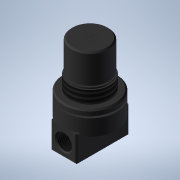
# Autodesk Inventor part: AP100-02_BODY
Saved by Autodesk Inventor 2021 (Build 250183000, 183)
## iProperties
Created: 2026-06-25
Part Number: AP100-02_BODY
Material: Generic
Catalog Web Link: www.3dfindit.com
Description: AP100 BODY-Pressure Control Valve
Vendor: SMC
Document SubType Name: Modeling
Designer: psAdmin
Manufacturer: SMC
Mass: 54.57 g
Surface Area: 113.774 cm^2
Volume: 54.57 cm^3
Density: 1 g/cm^3
Appearance: PSOLRGB-176-176-176
Category: PARTsolutions
Company: SMC
Title: AP100-02_BODY
Author: Cadenas PARTsolutions
Comments: Pressure Control Valve
PSOL_IDENT_0: {$CADENAS_DATA/23d-libs/smc_jp/air_line_equipment/pressure_control_equipment/pressure_control_valve/
PSOL_IDENT_1: parts/ap100_body.prj},187 {VTYP=3D},{NB=AP100-02_BODY},{LINA=AP100-02_BODY},{NN=AP100 BODY},{DATE=25
PSOL_IDENT_2: .06.2026 06:59:34},{GEOMDATE=28.10.2020 06:44:50},{VERSION=},{LINEID=10},{WBVAR=THREAD2,ACCESSORY},{
PSOL_IDENT_3: WBNUMERIC=}  {NB=AP100-02_BODY},{LINA=AP100-02_BODY},{KT=DUMMY},{THREAD2=02},{ACCESSORY=},{ORDER=AP1
PSOL_IDENT_4: 00-02},{RA=13.157},{RD=11.6}
NB: AP100-02_BODY
NN: AP100 BODY
NT: Pressure Control Valve
NBSYN: $ORDER._BODY
LINA: AP100-02_BODY
CATALOG: SMC (JP
THREAD2: (02) 1/4
ACCESSORY: (-) None
SUPPLIER: SMC
ARTICLENO: AP100-02_BODY
BOMINFO: AP100-02_BODY
CREATOR: CADENAS GmbH
Autodesk Inventor part; units mm, degrees
sketch "Sketch_1" plane through (0, 0, 0) normal (0, 0, 1) x (1, 0, 0)
  line L0 (-10, 10) -> (-10, -9)
  line L1 (-10, -9) -> (-9, -10)
  line L2 (-9, -10) -> (9, -10)
  line L3 (9, -10) -> (10, -9)
  line L4 (10, -9) -> (10, 10)
  line L5 (10, 10) -> (-10, 10)
  constraints: 12 end point
extrude "Extrusion1" add sketch "Sketch_1" along normal mid plane 40
sketch "Sketch_2" plane through (0, 0, 0) normal (0, 1, 0) x (-1, 0, 0)
  line L0 (15, 25) -> (-15, 25)
  line L1 (-15, 25) -> (-15, -25)
  line L2 (-15, -25) -> (15, -25)
  line L3 (15, -25) -> (15, 25)
  line L4 (10, -19) -> (10, 19)
  line L5 (10, 19) -> (9, 20)
  line L6 (9, 20) -> (-9, 20)
  line L7 (-9, 20) -> (-10, 19)
  line L8 (-10, 19) -> (-10, -19)
  line L9 (-10, -19) -> (-9, -20)
  line L10 (-9, -20) -> (9, -20)
  line L11 (9, -20) -> (10, -19)
  constraints: 24 end point
extrude "Extrusion2" cut sketch "Sketch_2" along normal mid plane 40
sketch "Sketch_3" plane through (0, 0, 0) normal (1, 0, 0) x (0, 1, 0)
  line L0 (15, 25) -> (-15, 25)
  line L1 (-15, 25) -> (-15, -25)
  line L2 (-15, -25) -> (15, -25)
  line L3 (15, -25) -> (15, -20)
  line L4 (15, -20) -> (-9, -20)
  line L5 (-9, -20) -> (-10, -19)
  line L6 (-10, -19) -> (-10, 19)
  line L7 (-10, 19) -> (-9, 20)
  line L8 (-9, 20) -> (15, 20)
  line L9 (15, 20) -> (15, 25)
  constraints: 20 end point
extrude "Extrusion3" cut sketch "Sketch_3" along normal mid plane 20
sketch "Sketch_4" plane through (0, 0, 0) normal (0, 0, 1) x (1, 0, 0)
  line L0 (0, 59) -> (0, 8)
  line L1 (0, 8) -> (-20, 8)
  line L2 (-20, 8) -> (-20, 20)
  line L3 (-20, 20) -> (-18, 20)
  line L4 (-18, 20) -> (-18, 21.5)
  line L5 (-18, 21.5) -> (-20, 21.5)
  line L6 (-20, 21.5) -> (-20, 24.5)
  line L7 (-20, 24.5) -> (-19, 25.5)
  line L8 (-19, 25.5) -> (-15, 25.5)
  line L9 (-15, 25.5) -> (-15, 35)
  line L10 (-15, 35) -> (-14, 35)
  line L11 (-14, 35) -> (-14, 36)
  line L12 (-14, 36) -> (-12, 36)
  line L13 (-12, 36) -> (-12, 37.09)
  line L14 (-12, 37.09) -> (-14, 37.09)
  line L15 (-14, 37.09) -> (-14, 58)
  line L16 (-14, 58) -> (-13, 59)
  line L17 (-13, 59) -> (0, 59)
  line L18 (0, 59) -> (0, 8)
  constraints: 38 end point
revolve "Revolution1" add sketch "Sketch_4" angle 360 about axis through (0, 59, 0) along (0, 1, 0)
thread "Thread1" size "M30x3.5" class "6g" standard "ISO Metric profile" full length
sketch "Sketch_5" plane through (0, 0, 0) normal (1, 0, 0) x (0, 1, 0)
  line L0 (0, 20) -> (0, 5.0961)
  line L1 (0, 5.0961) -> (-5.7225, 8.4)
  line L2 (-5.7225, 8.4) -> (-5.7225, 19.144)
  line L3 (-5.7225, 19.144) -> (-6.5785, 20)
  line L4 (-6.5785, 20) -> (0, 20)
  line L5 (0, 20) -> (0, 5.0961)
  constraints: 12 end point
revolve "Revolution2" cut sketch "Sketch_5" angle 360 about axis through (0, 0, 20) along (0, 0, 1)
thread "Thread2" size "G13.157x1.337" designation "G 1/4" standard "ISO Pipe Threads" full length
sketch "Sketch_6" plane through (0, 0, 0) normal (1, 0, 0) x (0, 1, 0)
  line L0 (0, -5.0961) -> (0, -20)
  line L1 (0, -20) -> (-6.5785, -20)
  line L2 (-6.5785, -20) -> (-5.7225, -19.144)
  line L3 (-5.7225, -19.144) -> (-5.7225, -8.4)
  line L4 (-5.7225, -8.4) -> (0, -5.0961)
  line L5 (0, -5.0961) -> (0, -20)
  constraints: 12 end point
revolve "Revolution3" cut sketch "Sketch_6" angle 360 about axis through (0, 0, -5.0961) along (0, 0, 1)
thread "Thread3" size "G13.157x1.337" designation "G 1/4" standard "ISO Pipe Threads" full length
sketch "Sketch_10" plane through (0, 59, 0) normal (0, 1, 0) x (1, 0, 0)
  line L0 (-3, -0.5) -> (-1, -0.5)
  arc A0 (-0.5, -1) -> (-1, -0.5) centre (-1, -1) ccw
  line L1 (-0.5, -1) -> (-0.5, -3)
  line L2 (-0.5, -3) -> (0.5, -3)
  line L3 (0.5, -3) -> (0.5, -1)
  arc A1 (1, -0.5) -> (0.5, -1) centre (1, -1) ccw
  line L4 (1, -0.5) -> (3, -0.5)
  line L5 (3, -0.5) -> (3, 0.5)
  line L6 (3, 0.5) -> (1, 0.5)
  arc A2 (0.5, 1) -> (1, 0.5) centre (1, 1) ccw
  line L7 (0.5, 1) -> (0.5, 3)
  line L8 (0.5, 3) -> (-0.5, 3)
  line L9 (-0.5, 3) -> (-0.5, 1)
  arc A3 (-1, 0.5) -> (-0.5, 1) centre (-1, 1) ccw
  line L10 (-1, 0.5) -> (-3, 0.5)
  line L11 (-3, 0.5) -> (-3, -0.5)
  constraints: 24 end point, 8 point on circle, 4 centre point
extrude "Extrusion4" cut sketch "Sketch_10" against normal blind 0.2
sketch "Sketch_11" plane through (0, 59, 0) normal (0, 1, 0) x (1, 0, 0)
  circle A0 centre (0, 0) radius 4.1
  circle A1 centre (0, 0) radius 4
  constraints: 2 centre point
extrude "Extrusion5" cut sketch "Sketch_11" against normal blind 1
ref_plane "body_dummy_XY" through (0, 0, 0) normal (0, 0, -1) x (1, 0, 0)
ref_plane "body_dummy_YZ" through (0, 0, 0) normal (1, 0, 0) x (0, -1, 0)
ref_plane "body_dummy_ZX" through (0, 0, 0) normal (0, -1, 0) x (0, 0, -1)
ref_plane "body_nut_XY" through (0, 27.1, 0) normal (0, 1, 0) x (1, 0, 0)
ref_plane "body_nut_YZ" through (0, 27.1, 0) normal (1, 0, 0) x (0, 0, -1)
ref_plane "body_nut_ZX" through (0, 27.1, 0) normal (0, 0, -1) x (0, 1, 0)
body "Solid1"
